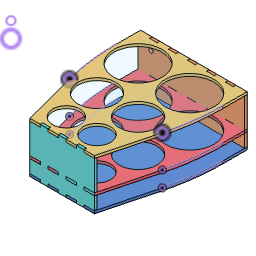
Zip Ties Peg Board Holder Laser Cut Version v5 (Autodesk Fusion 360 design; units mm, degrees)
Autodesk Fusion 360 part; units mm, degrees
sketch "Sketch1" plane through (0, 0, 0) normal (0, 1, 0) x (1, 0, 0) in component "Top Part"
  line L0 (0, 0) -> (24.5, 0) construction
  circle A0 centre (24.5, 0) radius 22.5
  line L1 (0, 0) -> (0, 91) construction
  circle A1 centre (30.75, 55.25) radius 28.75
  circle A2 centre (18.25, -42.75) radius 16.25
  line L2 (0, -66) -> (38.5, -66)
  line L3 (0, 91) -> (63.5, 91)
  line L4 (63.5, 91) -> (63.5, 29.5)
  line L5 (38.5, -66) -> (63.5, 29.5)
  line L6 (0, 91) -> (-63.5, 91)
  line L7 (-63.5, 91) -> (-63.5, 29.5)
  line L8 (-38.5, -66) -> (-63.5, 29.5)
  line L9 (0, -66) -> (-38.5, -66)
  circle A3 centre (-30.75, 55.25) radius 28.75
  circle A4 centre (-24.5, 0) radius 22.5
  circle A5 centre (-18.25, -42.75) radius 16.25
  line L10 (40.8333, 91) -> (49.8333, 91)
  line L11 (49.8333, 91) -> (49.8333, 88)
  line L12 (49.8333, 88) -> (40.8333, 88)
  line L13 (40.8333, 88) -> (40.8333, 91)
  line L14 (27.1667, 91) -> (18.1667, 91)
  line L15 (18.1667, 91) -> (18.1667, 88)
  line L16 (18.1667, 88) -> (27.1667, 88)
  line L17 (27.1667, 88) -> (27.1667, 91)
  line L18 (27.1667, 89.5) -> (40.8333, 89.5) construction
  line L19 (0, 91) -> (4.5, 91)
  line L20 (4.5, 91) -> (4.5, 88)
  line L21 (4.5, 88) -> (0, 88)
  line L22 (4.5, 89.5) -> (18.1667, 89.5) construction
  line L23 (49.8333, 89.5) -> (63.5, 89.5) construction
  line L24 (-49.8333, 91) -> (-49.8333, 88)
  line L25 (-49.8333, 88) -> (-40.8333, 88)
  line L26 (-40.8333, 88) -> (-40.8333, 91)
  line L27 (-27.1667, 88) -> (-27.1667, 91)
  line L28 (-18.1667, 88) -> (-27.1667, 88)
  line L29 (-18.1667, 91) -> (-18.1667, 88)
  line L30 (-4.5, 91) -> (-4.5, 88)
  line L31 (-4.5, 88) -> (0, 88)
  line L32 (0, -66) -> (4.5, -66)
  line L33 (4.5, -66) -> (4.5, -63)
  line L34 (4.5, -63) -> (0, -63)
  line L35 (17, -66) -> (26, -66)
  line L36 (26, -66) -> (26, -63)
  line L37 (26, -63) -> (17, -63)
  line L38 (17, -63) -> (17, -66)
  line L39 (38.5, -66) -> (38.5, -62) construction
  line L40 (26, -64.5) -> (38.5, -64.5) construction
  line L41 (17, -64.5) -> (4.5, -64.5) construction
  line L42 (-26, -66) -> (-26, -63)
  line L43 (-26, -63) -> (-17, -63)
  line L44 (-17, -63) -> (-17, -66)
  line L45 (-4.5, -66) -> (-4.5, -63)
  line L46 (-4.5, -63) -> (0, -63)
  dimension "d6" = 24.5
  dimension "d7" = 45
  dimension "d8" = 57.5
  dimension "d9" = 55.25
  dimension "d10" = 30.75
  dimension "d11" = 32.5
  dimension "d12" = 42.75
  dimension "d13" = 18.25
  dimension "d14" = 23.25
  dimension "d15" = 38.5
  dimension "d16" = 63.5
  dimension "d17" = 35.75
  dimension "d18" = 61.5
  dimension "d21" = 3
  dimension "d22" = 9
  dimension "d23" = 9
  dimension "d24" = 3
  dimension "d25" = 4.5
  dimension "d26" = 3
  dimension "d27" = 4.5
  dimension "d28" = 3
  dimension "d29" = 3
  dimension "d30" = 9
  constraint coincident L0.start L1.start
  constraint horizontal L0
  constraint coincident L0.end A0.centre
  constraint perpendicular L0 L1
  constraint horizontal L2
  constraint horizontal L3
  constraint perpendicular L3 L4
  constraint symmetric A0 L1 A4
  constraint symmetric L1 A1 A3
  constraint symmetric L1 A2 A5
  constraint symmetric L1 L2.start L9.start
  constraint symmetric L1 L2.end L8.start
  constraint symmetric L1 L3.start L6.start
  constraint symmetric L1 L3.end L6.end
  constraint symmetric L1 L4.end L7.end
  constraint horizontal L10
  constraint vertical L11
  constraint horizontal L12
  constraint vertical L13
  constraint coincident L3 L10.start
  constraint horizontal L14
  constraint vertical L15
  constraint horizontal L16
  constraint vertical L17
  constraint coincident L3 L14.start
  constraint coincident L1.end L3.start
  constraint midpoint L17 L18.start
  constraint midpoint L13 L18.end
  constraint horizontal L19
  constraint vertical L20
  constraint horizontal L21
  constraint midpoint L20 L22.start
  constraint midpoint L15 L22.end
  constraint midpoint L11 L23.start
  constraint coincident L4 L23.end
  constraint perpendicular L4 L23
  constraint equal L18 L23
  constraint equal L18 L22
  constraint symmetric L1 L10.start L26.end
  constraint symmetric L1 L10.end L24.start
  constraint symmetric L1 L11.end L24.end
  constraint symmetric L1 L12.end L25.end
  constraint symmetric L1 L14.start L27.end
  constraint symmetric L1 L14.end L29.start
  constraint symmetric L1 L15.end L28.start
  constraint symmetric L1 L16.end L27.start
  constraint symmetric L1 L19.end L30.start
  constraint symmetric L1 L20.end L30.end
  constraint symmetric L1 L21.end L31.end
  constraint coincident L2.start L9.start
  constraint horizontal L32
  constraint vertical L33
  constraint horizontal L34
  constraint horizontal L35
  constraint vertical L36
  constraint horizontal L37
  constraint vertical L38
  constraint coincident L2 L35.start
  constraint perpendicular L2 L39
  constraint midpoint L36 L40.start
  constraint coincident L39 L40.end
  constraint perpendicular L39 L40
  constraint midpoint L38 L41.start
  constraint midpoint L33 L41.end
  constraint equal L40 L41
  constraint symmetric L1 L32.end L45.start
  constraint symmetric L1 L33.end L45.end
  constraint symmetric L1 L34.end L46.end
  constraint symmetric L1 L35.start L44.end
  constraint symmetric L1 L35.end L42.start
  constraint symmetric L1 L36.end L42.end
  constraint symmetric L1 L37.end L43.end
  measures "d6" distance of L0.start L0.end
  measures "d7" diameter of A0
  measures "d8" diameter of A1
  measures "d9" vertical distance of L0.end A1.centre
  measures "d10" distance of L1 A1.centre
  measures "d11" diameter of A2
  measures "d12" vertical distance of L0.end A2.centre
  measures "d13" distance of L1 A2.centre
  measures "d14" distance of A2.centre L2
  measures "d15" distance of L2.start L2.end
  measures "d16" distance of L1.end L3.end
  measures "d17" distance of A1.centre L3
  measures "d18" distance of L3.end L4.end
  measures "d21" distance of L3 L12
  measures "d22" distance of L11.end L12.end
  measures "d23" distance of L15.end L16.end
  measures "d24" distance of L14 L16
  measures "d25" distance of L1 L20
  measures "d26" distance of L19 L21
  measures "d27" distance of L33.end L34.end
  measures "d28" distance of L32.end L33.end
  measures "d29" distance of L35.start L37.end
  measures "d30" distance of L36.end L37.end
extrude "Extrude1" add sketch "Sketch1" along normal blind 3 contours L2 L3 L4 L5 L6 L7 L8 L9 L11 L12 L13 L15 L16 L17 L20 L21 L24 L25 L26 L27 L28 L29 L30 L31 L33 L34 L36 L37 L38 L42 L43 L44 L45 L46 makes body 1 in component "Top Part"
sketch "Sketch1 (2)" plane through (0, 0, 66) normal (0, 0, 1) x (1, 0, 0) in component "Front Part"
  line L0 (-38.5, 0) -> (-26, 0)
  line L1 (-26, 0) -> (-26, 3)
  line L2 (-26, 3) -> (-38.5, 3)
  line L3 (-38.5, 3) -> (-38.5, 0)
  line L4 (-26, 0) -> (-17, 0)
  line L5 (-26, 0) -> (-17, 0)
  line L6 (-17, 0) -> (-17, 3)
  line L7 (-17, 3) -> (-26, 3)
  line L8 (-26, 3) -> (-26, 0)
  line L9 (-17, 0) -> (-4.5, 0)
  line L10 (-4.5, 0) -> (-4.5, 3)
  line L11 (-4.5, 3) -> (-17, 3)
  line L12 (-17, 3) -> (-17, 0)
  line L13 (-4.5, 3) -> (4.5, 3)
  line L14 (-4.5, 0) -> (4.5, 0)
  line L15 (4.5, 0) -> (4.5, 3)
  line L16 (4.5, 3) -> (-4.5, 3)
  line L17 (-4.5, 3) -> (-4.5, 0)
  line L18 (4.5, 3) -> (17, 3)
  line L19 (4.5, 0) -> (17, 0)
  line L20 (17, 0) -> (17, 3)
  line L21 (17, 3) -> (4.5, 3)
  line L22 (4.5, 3) -> (4.5, 0)
  line L23 (26, 0) -> (17, 0)
  line L24 (17, 0) -> (26, 0)
  line L25 (26, 0) -> (26, 3)
  line L26 (26, 3) -> (17, 3)
  line L27 (17, 3) -> (17, 0)
  line L28 (26, 0) -> (38.5, 0)
  line L29 (38.5, 0) -> (38.5, 3)
  line L30 (38.5, 3) -> (26, 3)
  line L31 (26, 3) -> (26, 0)
  line L32 (-38.5, 3) -> (38.5, 3)
  line L33 (38.5, 3) -> (38.5, -57)
  line L34 (38.5, -57) -> (-38.5, -57)
  line L35 (-38.5, -57) -> (-38.5, 3)
  line L36 (-38.5, -27) -> (38.5, -27) construction
  line L37 (-38.5, -54) -> (-26, -54)
  line L38 (-26, -54) -> (-26, -57)
  line L39 (-17, -57) -> (-17, -54)
  line L40 (-17, -54) -> (-4.5, -54)
  line L41 (-4.5, -54) -> (-4.5, -57)
  line L42 (4.5, -57) -> (4.5, -54)
  line L43 (4.5, -54) -> (17, -54)
  line L44 (17, -57) -> (17, -54)
  line L45 (26, -54) -> (26, -57)
  line L46 (26, -54) -> (38.5, -54)
  dimension "d33" = 60
  constraint horizontal L32
  constraint vertical L33
  constraint horizontal L34
  constraint vertical L35
  constraint coincident L2.end L3.start
  constraint coincident L29.end L33
  constraint midpoint L35 L36.start
  constraint midpoint L33 L36.end
  constraint symmetric L0.start L36 L37.start
  constraint symmetric L0.end L36 L37.end
  constraint symmetric L1.end L36 L38.end
  constraint symmetric L4.end L36 L39.end
  constraint symmetric L9.end L36 L40.end
  constraint symmetric L10.end L36 L41.end
  constraint symmetric L6.end L36 L39.start
  constraint symmetric L14.end L36 L42.end
  constraint symmetric L19.end L36 L43.end
  constraint symmetric L13.end L36 L42.start
  constraint symmetric L23.start L36 L45.start
  constraint symmetric L25.end L36 L45.end
  constraint symmetric L18.end L36 L44.start
  constraint symmetric L28.end L36 L46.end
  measures "d33" distance of L29.end L33.end
extrude "Extrude1'" add sketch "Sketch1 (2)" against normal blind 3 separate body contours L0 L4 L5 L9 L14 L19 L23 L24 L28 L33 L34 L35 L37 L38 L39 L40 L41 L42 L43 L44 L45 L46 | L1 L4 L5 L6 L7 L8 L12 L32 | L10 L13 L14 L15 L16 L17 L22 L32 | L20 L23 L24 L25 L26 L27 L31 L32 makes body 2 in component "Front Part"
sketch "Sketch1 (3)" plane through (0, 0, -91) normal (0, 0, -1) x (-1, 0, 0) in component "Back Part"
  line L0 (-18.1667, 0) -> (-4.5, 0)
  line L1 (-4.5, 0) -> (-4.5, 3)
  line L2 (-4.5, 3) -> (-18.1667, 3)
  line L3 (-18.1667, 3) -> (-18.1667, 0)
  line L4 (-63.5, 0) -> (-49.8333, 0)
  line L5 (-49.8333, 0) -> (-49.8333, 3)
  line L6 (-49.8333, 3) -> (-63.5, 3)
  line L7 (-63.5, 3) -> (-63.5, 0)
  line L8 (-49.8333, 0) -> (-40.8333, 0)
  line L9 (-40.8333, 0) -> (-40.8333, 3)
  line L10 (-40.8333, 3) -> (-49.8333, 3)
  line L11 (-49.8333, 3) -> (-49.8333, 0)
  line L12 (-40.8333, 0) -> (-27.1667, 0)
  line L13 (-27.1667, 0) -> (-27.1667, 3)
  line L14 (-27.1667, 3) -> (-40.8333, 3)
  line L15 (-40.8333, 3) -> (-40.8333, 0)
  line L16 (-27.1667, 0) -> (-18.1667, 0)
  line L17 (-18.1667, 0) -> (-18.1667, 3)
  line L18 (-18.1667, 3) -> (-27.1667, 3)
  line L19 (-27.1667, 3) -> (-27.1667, 0)
  line L20 (-4.5, 0) -> (4.5, 0)
  line L21 (4.5, 0) -> (4.5, 3)
  line L22 (4.5, 3) -> (-4.5, 3)
  line L23 (-4.5, 3) -> (-4.5, 0)
  line L24 (4.5, 0) -> (18.1667, 0)
  line L25 (18.1667, 0) -> (18.1667, 3)
  line L26 (18.1667, 3) -> (4.5, 3)
  line L27 (4.5, 3) -> (4.5, 0)
  line L28 (18.1667, 0) -> (27.1667, 0)
  line L29 (27.1667, 0) -> (27.1667, 3)
  line L30 (27.1667, 3) -> (18.1667, 3)
  line L31 (18.1667, 3) -> (18.1667, 0)
  line L32 (27.1667, 0) -> (40.8333, 0)
  line L33 (40.8333, 0) -> (40.8333, 3)
  line L34 (40.8333, 3) -> (27.1667, 3)
  line L35 (27.1667, 3) -> (27.1667, 0)
  line L36 (40.8333, 0) -> (49.8333, 0)
  line L37 (49.8333, 0) -> (49.8333, 3)
  line L38 (49.8333, 3) -> (40.8333, 3)
  line L39 (40.8333, 3) -> (40.8333, 0)
  line L40 (49.8333, 0) -> (63.5, 0)
  line L41 (63.5, 0) -> (63.5, 3)
  line L42 (63.5, 3) -> (49.8333, 3)
  line L43 (49.8333, 3) -> (49.8333, 0)
  line L44 (-63.5, 3) -> (63.5, 3)
  line L45 (63.5, 3) -> (63.5, -57)
  line L46 (63.5, -57) -> (-63.5, -57)
  line L47 (-63.5, -57) -> (-63.5, 3)
  line L48 (-63.5, -27) -> (63.5, -27) construction
  line L49 (-63.5, -54) -> (-49.8333, -54)
  line L50 (-49.8333, -54) -> (-49.8333, -57)
  line L51 (-40.8333, -54) -> (-40.8333, -57)
  line L52 (-40.8333, -54) -> (-27.1667, -54)
  line L53 (-27.1667, -57) -> (-27.1667, -54)
  line L54 (-18.1667, -57) -> (-18.1667, -54)
  line L55 (-18.1667, -54) -> (-4.5, -54)
  line L56 (-4.5, -57) -> (-4.5, -54)
  line L57 (4.5, -54) -> (4.5, -57)
  line L58 (4.5, -54) -> (18.1667, -54)
  line L59 (18.1667, -57) -> (18.1667, -54)
  line L60 (27.1667, -54) -> (27.1667, -57)
  line L61 (27.1667, -54) -> (40.8333, -54)
  line L62 (40.8333, -57) -> (40.8333, -54)
  line L63 (49.8333, -54) -> (49.8333, -57)
  line L64 (49.8333, -54) -> (63.5, -54)
  circle A0 centre (-48, -9) radius 2.5
  line L65 (-26, -54) -> (-26, -57)
  line L66 (-26, -57) -> (-17, -57)
  line L67 (-17, -57) -> (-17, -54)
  line L68 (-17, -54) -> (-4.5, -54)
  line L69 (-4.5, -54) -> (-4.5, -57)
  line L70 (-4.5, -57) -> (4.5, -57)
  line L71 (4.5, -57) -> (4.5, -54)
  line L72 (4.5, -54) -> (17, -54)
  line L73 (17, -54) -> (17, -57)
  line L74 (17, -57) -> (26, -57)
  line L75 (26, -57) -> (26, -54)
  line L76 (26, -54) -> (38.5, -54)
  line L77 (38.5, -54) -> (38.5, 0)
  line L78 (38.5, 0) -> (26, 0)
  line L79 (26, 0) -> (26, 3)
  line L80 (26, 3) -> (17, 3)
  line L81 (17, 3) -> (17, 0)
  line L82 (17, 0) -> (4.5, 0)
  line L83 (4.5, 0) -> (4.5, 3)
  line L84 (4.5, 3) -> (-4.5, 3)
  line L85 (-4.5, 3) -> (-4.5, 0)
  line L86 (-4.5, 0) -> (-17, 0)
  line L87 (-17, 0) -> (-17, 3)
  line L88 (-17, 3) -> (-26, 3)
  line L89 (-26, 3) -> (-26, 0)
  line L90 (-26, 0) -> (-38.5, 0)
  line L91 (-38.5, 0) -> (-38.5, -54)
  line L92 (-38.5, -54) -> (-26, -54)
  circle A1 centre (48, -9) radius 2.5
  line L93 (48, -9) -> (63.5, -9) construction
  line L94 (-48, -9) -> (-63.5, -9) construction
  circle A2 centre (-48, -45) radius 2.5
  circle A3 centre (48, -45) radius 2.5
  dimension "d36" = 60
  dimension "d46" = 5
  dimension "d48" = 5
  dimension "d49" = 96
  dimension "d50" = 36
  constraint horizontal L44
  constraint vertical L45
  constraint horizontal L46
  constraint vertical L47
  constraint coincident L6.end L7.start
  constraint coincident L41.end L45
  constraint midpoint L47 L48.start
  constraint midpoint L45 L48.end
  constraint symmetric L0.start L48 L54.end
  constraint symmetric L0.end L48 L55.end
  constraint symmetric L2.end L48 L54.start
  constraint symmetric L4.start L48 L49.start
  constraint symmetric L4.end L48 L49.end
  constraint symmetric L5.end L48 L50.end
  constraint symmetric L8.end L48 L51.start
  constraint symmetric L9.end L48 L51.end
  constraint symmetric L12.end L48 L52.end
  constraint symmetric L13.end L48 L53.start
  constraint symmetric L20.end L48 L57.start
  constraint symmetric L21.end L48 L57.end
  constraint symmetric L1.end L48 L56.start
  constraint symmetric L24.end L48 L58.end
  constraint symmetric L28.end L48 L60.start
  constraint symmetric L29.end L48 L60.end
  constraint symmetric L25.end L48 L59.start
  constraint symmetric L32.end L48 L61.end
  constraint symmetric L36.end L48 L63.start
  constraint symmetric L37.end L48 L63.end
  constraint symmetric L33.end L48 L62.start
  constraint symmetric L40.end L48 L64.end
  constraint coincident A1.centre L93.start
  constraint coincident L45 L93.end
  constraint perpendicular L45 L93
  constraint coincident A0.centre L94.start
  constraint coincident L47 L94.end
  constraint perpendicular L47 L94
  constraint collinear L93 L94
  constraint equal L93 L94
  constraint symmetric L48 A0 A2
  constraint symmetric L48 A1 A3
  measures "d36" distance of L41.end L45.end
  measures "d46" diameter of A0
  measures "d48" diameter of A1
  measures "d49" distance of A0.centre A1.centre
  measures "d50" distance of A1.centre A3.centre
extrude "Extrude1''" add sketch "Sketch1 (3)" against normal blind 3 separate body contours L3 L16 L17 L18 L44 L88 L89 | L0 L12 L16 L20 L24 L28 L32 L46 L52 L54 L55 L56 L57 L58 L59 L61 L65 L66 L68 L69 L70 L71 L72 L74 L75 L76 L77 L78 L82 L86 L90 L91 L92 | L13 L16 L18 L19 L44 L89 L90 | L1 L20 L21 L22 L23 L27 L44 L83 L84 L85 | L4 L8 L12 L46 L47 L49 L50 L51 L52 L91 | L5 L8 L9 L10 L11 L15 L44 | L25 L28 L30 L31 L44 L79 L80 | L46 L53 L65 L92 | L28 L29 L30 L35 L44 L78 L79 | L32 L36 L40 L45 L46 L61 L62 L63 L64 L77 | L33 L36 L37 L38 L39 L43 L44 | L46 L60 L75 L76 makes body 3 in component "Back Part"
sketch "Sketch1 (4)" plane through (0, -57, 0) normal (0, -1, 0) x (1, 0, 0) in component "Bottom Part"
  line L0 (40.8333, -91) -> (49.8333, -91)
  line L1 (49.8333, -91) -> (49.8333, -88)
  line L2 (49.8333, -88) -> (40.8333, -88)
  line L3 (40.8333, -88) -> (40.8333, -91)
  line L4 (49.8333, -91) -> (63.5, -91)
  line L5 (63.5, -91) -> (63.5, -88)
  line L6 (63.5, -88) -> (49.8333, -88)
  line L7 (49.8333, -88) -> (49.8333, -91)
  line L8 (27.1667, -91) -> (40.8333, -91)
  line L9 (40.8333, -91) -> (40.8333, -88)
  line L10 (40.8333, -88) -> (27.1667, -88)
  line L11 (27.1667, -88) -> (27.1667, -91)
  line L12 (18.1667, -91) -> (27.1667, -91)
  line L13 (27.1667, -91) -> (27.1667, -88)
  line L14 (27.1667, -88) -> (18.1667, -88)
  line L15 (18.1667, -88) -> (18.1667, -91)
  line L16 (4.5, -91) -> (18.1667, -91)
  line L17 (18.1667, -91) -> (18.1667, -88)
  line L18 (18.1667, -88) -> (4.5, -88)
  line L19 (4.5, -88) -> (4.5, -91)
  line L20 (-4.5, -91) -> (4.5, -91)
  line L21 (4.5, -91) -> (4.5, -88)
  line L22 (4.5, -88) -> (-4.5, -88)
  line L23 (-4.5, -88) -> (-4.5, -91)
  line L24 (-18.1667, -91) -> (-4.5, -91)
  line L25 (-4.5, -91) -> (-4.5, -88)
  line L26 (-4.5, -88) -> (-18.1667, -88)
  line L27 (-18.1667, -88) -> (-18.1667, -91)
  line L28 (-27.1667, -91) -> (-18.1667, -91)
  line L29 (-18.1667, -91) -> (-18.1667, -88)
  line L30 (-18.1667, -88) -> (-27.1667, -88)
  line L31 (-27.1667, -88) -> (-27.1667, -91)
  line L32 (-40.8333, -91) -> (-27.1667, -91)
  line L33 (-27.1667, -91) -> (-27.1667, -88)
  line L34 (-27.1667, -88) -> (-40.8333, -88)
  line L35 (-40.8333, -88) -> (-40.8333, -91)
  line L36 (-49.8333, -91) -> (-40.8333, -91)
  line L37 (-40.8333, -91) -> (-40.8333, -88)
  line L38 (-40.8333, -88) -> (-49.8333, -88)
  line L39 (-49.8333, -88) -> (-49.8333, -91)
  line L40 (-63.5, -91) -> (-49.8333, -91)
  line L41 (-49.8333, -91) -> (-49.8333, -88)
  line L42 (-49.8333, -88) -> (-63.5, -88)
  line L43 (-63.5, -88) -> (-63.5, -91)
  circle A0 centre (24.5, 0) radius 22.5
  circle A1 centre (-30.75, -55.25) radius 28.75
  circle A2 centre (-24.5, 0) radius 22.5
  circle A3 centre (30.75, -55.25) radius 28.75
  circle A4 centre (-18.25, 42.75) radius 16.25
  circle A5 centre (18.25, 42.75) radius 16.25
  line L44 (-4.5, 63) -> (-4.5, 66)
  line L45 (-4.5, 66) -> (-17, 66)
  line L46 (-17, 66) -> (-17, 63)
  line L47 (-17, 63) -> (-26, 63)
  line L48 (-26, 63) -> (-26, 66)
  line L49 (-26, 66) -> (-38.5, 66)
  line L50 (-38.5, 66) -> (-63.5, -29.5)
  line L51 (-63.5, -29.5) -> (-63.5, -91)
  line L52 (-63.5, -91) -> (-49.8333, -91)
  line L53 (-49.8333, -91) -> (-49.8333, -88)
  line L54 (-49.8333, -88) -> (-40.8333, -88)
  line L55 (-40.8333, -88) -> (-40.8333, -91)
  line L56 (-40.8333, -91) -> (-27.1667, -91)
  line L57 (-27.1667, -91) -> (-27.1667, -88)
  line L58 (-27.1667, -88) -> (-18.1667, -88)
  line L59 (-18.1667, -88) -> (-18.1667, -91)
  line L60 (-18.1667, -91) -> (-4.5, -91)
  line L61 (-4.5, -91) -> (-4.5, -88)
  line L62 (-4.5, -88) -> (4.5, -88)
  line L63 (4.5, -88) -> (4.5, -91)
  line L64 (4.5, -91) -> (18.1667, -91)
  line L65 (18.1667, -91) -> (18.1667, -88)
  line L66 (18.1667, -88) -> (27.1667, -88)
  line L67 (27.1667, -88) -> (27.1667, -91)
  line L68 (27.1667, -91) -> (40.8333, -91)
  line L69 (40.8333, -91) -> (40.8333, -88)
  line L70 (40.8333, -88) -> (49.8333, -88)
  line L71 (49.8333, -88) -> (49.8333, -91)
  line L72 (49.8333, -91) -> (63.5, -91)
  line L73 (63.5, -91) -> (63.5, -29.5)
  line L74 (63.5, -29.5) -> (38.5, 66)
  line L75 (38.5, 66) -> (26, 66)
  line L76 (26, 66) -> (26, 63)
  line L77 (26, 63) -> (17, 63)
  line L78 (17, 63) -> (17, 66)
  line L79 (17, 66) -> (4.5, 66)
  line L80 (4.5, 66) -> (4.5, 63)
  line L81 (4.5, 63) -> (-4.5, 63)
  line L82 (26, 66) -> (38.5, 66)
  line L83 (38.5, 66) -> (26, 66)
  line L84 (26, 66) -> (26, 63)
  line L85 (26, 63) -> (38.5, 63)
  line L86 (38.5, 63) -> (38.5, 66)
  line L87 (26, 66) -> (17, 66)
  line L88 (17, 66) -> (17, 63)
  line L89 (17, 63) -> (26, 63)
  line L90 (26, 63) -> (26, 66)
  line L91 (17, 66) -> (4.5, 66)
  line L92 (4.5, 66) -> (4.5, 63)
  line L93 (4.5, 63) -> (17, 63)
  line L94 (17, 63) -> (17, 66)
  line L95 (4.5, 66) -> (-4.5, 66)
  line L96 (-4.5, 66) -> (-4.5, 63)
  line L97 (-4.5, 63) -> (4.5, 63)
  line L98 (4.5, 63) -> (4.5, 66)
  line L99 (-4.5, 66) -> (-17, 66)
  line L100 (-17, 66) -> (-17, 63)
  line L101 (-17, 63) -> (-4.5, 63)
  line L102 (-4.5, 63) -> (-4.5, 66)
  line L103 (-17, 66) -> (-26, 66)
  line L104 (-26, 66) -> (-26, 63)
  line L105 (-26, 63) -> (-17, 63)
  line L106 (-17, 63) -> (-17, 66)
  line L107 (-26, 66) -> (-38.5, 66)
  line L108 (-38.5, 66) -> (-38.5, 63)
  line L109 (-38.5, 63) -> (-26, 63)
  line L110 (-26, 63) -> (-26, 66)
extrude "Extrude1'''" add sketch "Sketch1 (4)" against normal blind 3 separate body contours L3 L8 L9 L10 L11 L13 L67 L68 L69 | L1 L4 L5 L6 L7 L71 L72 L73 | L2 L6 L10 L14 L18 L22 L26 L30 L34 L38 L42 L47 L50 L51 L54 L58 L62 L66 L70 L73 L74 L77 L81 L85 L86 L89 L93 L97 L101 L105 L108 L109 | L15 L16 L17 L18 L19 L21 L63 L64 L65 | L23 L24 L25 L26 L27 L29 L59 L60 L61 | L75 L76 L82 L83 L84 L85 L86 L90 | L31 L32 L33 L34 L35 L37 L55 L56 L57 | L78 L79 L80 L88 L91 L92 L93 L94 L98 | L39 L40 L41 L42 L43 L51 L52 L53 | L44 L45 L46 L96 L99 L100 L101 L102 L106 | L48 L49 L104 L107 L108 L109 L110 | A0 | A1 | A2 | A3 | A4 | A5 makes body 4 in component "Bottom Part"
ref_plane "WorkPlane1" through (0, -37, -12.5) normal (0, -1, 0) x (1, 0, 0) in component "Middle Part"
sketch "Sketch1 (5)" plane through (0, -37, 0) normal (0, -1, 0) x (-1, 0, 0) in component "Middle Part"
  circle A0 centre (-24.5, 0) radius 22.5
  circle A1 centre (30.75, 55.25) radius 28.75
  circle A2 centre (24.5, 0) radius 22.5
  circle A3 centre (-30.75, 55.25) radius 28.75
  circle A4 centre (18.25, -42.75) radius 16.25
  circle A5 centre (-18.25, -42.75) radius 16.25
  line L0 (4.5, -63) -> (4.5, -66)
  line L1 (4.5, -66) -> (17, -66)
  line L2 (17, -66) -> (17, -63)
  line L3 (17, -63) -> (26, -63)
  line L4 (26, -63) -> (26, -66)
  line L5 (26, -66) -> (38.5, -66)
  line L6 (38.5, -66) -> (63.5, 29.5)
  line L7 (63.5, 29.5) -> (63.5, 91)
  line L8 (63.5, 91) -> (49.8333, 91)
  line L9 (49.8333, 91) -> (49.8333, 88)
  line L10 (49.8333, 88) -> (40.8333, 88)
  line L11 (40.8333, 88) -> (40.8333, 91)
  line L12 (40.8333, 91) -> (27.1667, 91)
  line L13 (27.1667, 91) -> (27.1667, 88)
  line L14 (27.1667, 88) -> (18.1667, 88)
  line L15 (18.1667, 88) -> (18.1667, 91)
  line L16 (18.1667, 91) -> (4.5, 91)
  line L17 (4.5, 91) -> (4.5, 88)
  line L18 (4.5, 88) -> (-4.5, 88)
  line L19 (-4.5, 88) -> (-4.5, 91)
  line L20 (-4.5, 91) -> (-18.1667, 91)
  line L21 (-18.1667, 91) -> (-18.1667, 88)
  line L22 (-18.1667, 88) -> (-27.1667, 88)
  line L23 (-27.1667, 88) -> (-27.1667, 91)
  line L24 (-27.1667, 91) -> (-40.8333, 91)
  line L25 (-40.8333, 91) -> (-40.8333, 88)
  line L26 (-40.8333, 88) -> (-49.8333, 88)
  line L27 (-49.8333, 88) -> (-49.8333, 91)
  line L28 (-49.8333, 91) -> (-63.5, 91)
  line L29 (-63.5, 91) -> (-63.5, 29.5)
  line L30 (-63.5, 29.5) -> (-38.5, -66)
  line L31 (-38.5, -66) -> (-26, -66)
  line L32 (-26, -66) -> (-26, -63)
  line L33 (-26, -63) -> (-17, -63)
  line L34 (-17, -63) -> (-17, -66)
  line L35 (-17, -66) -> (-4.5, -66)
  line L36 (-4.5, -66) -> (-4.5, -63)
  line L37 (-4.5, -63) -> (4.5, -63)
extrude "Extrude1''''" add sketch "Sketch1 (5)" along normal mid plane 3 separate body makes body 5 in component "Middle Part"
fillet "Fillet1" radius 252.5 2 edges at (-63.5, 1.5, -29.5) (63.5, 1.5, -29.5) on bodies 1 in component "Top Part"
fillet "Fillet1'" radius 252.5 2 edges at (-63.5, -37, -29.5) (63.5, -37, -29.5) on bodies 5 in component "Middle Part"
fillet "Fillet1''" radius 252.5 2 edges at (-63.5, -55.5, -29.5) (63.5, -55.5, -29.5) on bodies 4 in component "Bottom Part"
sketch "Front Part DXF" plane through (0, 0, 66) normal (0, 0, 1) x (1, 0, 0)
  line L0 (26, -57) -> (26, -54)
  line L1 (26, -54) -> (38.5, -54)
  line L2 (38.5, -54) -> (38.5, 0)
  line L3 (38.5, 0) -> (26, 0)
  line L4 (26, 0) -> (26, 3)
  line L5 (26, 3) -> (17, 3)
  line L6 (17, 3) -> (17, 0)
  line L7 (17, 0) -> (4.5, 0)
  line L8 (4.5, 0) -> (4.5, 3)
  line L9 (4.5, 3) -> (-4.5, 3)
  line L10 (-4.5, 3) -> (-4.5, 0)
  line L11 (-4.5, 0) -> (-17, 0)
  line L12 (-17, 0) -> (-17, 3)
  line L13 (-17, 3) -> (-26, 3)
  line L14 (-26, 3) -> (-26, 0)
  line L15 (-26, 0) -> (-38.5, 0)
  line L16 (-38.5, 0) -> (-38.5, -54)
  line L17 (-38.5, -54) -> (-26, -54)
  line L18 (-26, -54) -> (-26, -57)
  line L19 (-26, -57) -> (-17, -57)
  line L20 (-17, -57) -> (-17, -54)
  line L21 (-17, -54) -> (-4.5, -54)
  line L22 (-4.5, -54) -> (-4.5, -57)
  line L23 (-4.5, -57) -> (4.5, -57)
  line L24 (4.5, -57) -> (4.5, -54)
  line L25 (4.5, -54) -> (17, -54)
  line L26 (17, -54) -> (17, -57)
  line L27 (17, -57) -> (26, -57)
sketch "Top Part DXF" plane through (0, 3, 0) normal (0, 1, 0) x (-1, 0, 0)
  circle A0 centre (-24.5, 0) radius 22.5
  circle A1 centre (30.75, -55.25) radius 28.75
  circle A2 centre (24.5, 0) radius 22.5
  circle A3 centre (-30.75, -55.25) radius 28.75
  circle A4 centre (18.25, 42.75) radius 16.25
  circle A5 centre (-18.25, 42.75) radius 16.25
  line L0 (4.5, 66) -> (4.5, 63)
  line L1 (4.5, 63) -> (-4.5, 63)
  line L2 (-4.5, 63) -> (-4.5, 66)
  line L3 (-4.5, 66) -> (-17, 66)
  line L4 (-17, 66) -> (-17, 63)
  line L5 (-17, 63) -> (-26, 63)
  line L6 (-26, 63) -> (-26, 66)
  line L7 (-26, 66) -> (-38.5, 66)
  line L8 (-38.5, 66) -> (-55.2689, 1.9426)
  line L9 (-63.5, -62.0021) -> (-63.5, -91)
  line L10 (-63.5, -91) -> (-49.8333, -91)
  line L11 (-49.8333, -91) -> (-49.8333, -88)
  line L12 (-49.8333, -88) -> (-40.8333, -88)
  line L13 (-40.8333, -88) -> (-40.8333, -91)
  line L14 (-40.8333, -91) -> (-27.1667, -91)
  line L15 (-27.1667, -91) -> (-27.1667, -88)
  line L16 (-27.1667, -88) -> (-18.1667, -88)
  line L17 (-18.1667, -88) -> (-18.1667, -91)
  line L18 (-18.1667, -91) -> (-4.5, -91)
  line L19 (-4.5, -91) -> (-4.5, -88)
  line L20 (-4.5, -88) -> (4.5, -88)
  line L21 (4.5, -88) -> (4.5, -91)
  line L22 (4.5, -91) -> (18.1667, -91)
  line L23 (18.1667, -91) -> (18.1667, -88)
  line L24 (18.1667, -88) -> (27.1667, -88)
  line L25 (27.1667, -88) -> (27.1667, -91)
  line L26 (27.1667, -91) -> (40.8333, -91)
  line L27 (40.8333, -91) -> (40.8333, -88)
  line L28 (40.8333, -88) -> (49.8333, -88)
  line L29 (49.8333, -88) -> (49.8333, -91)
  line L30 (49.8333, -91) -> (63.5, -91)
  line L31 (63.5, -91) -> (63.5, -62.0021)
  line L32 (55.2689, 1.9426) -> (38.5, 66)
  line L33 (38.5, 66) -> (26, 66)
  line L34 (26, 66) -> (26, 63)
  line L35 (26, 63) -> (17, 63)
  line L36 (17, 63) -> (17, 66)
  line L37 (17, 66) -> (4.5, 66)
  arc A6 (-55.2689, 1.9426) -> (-63.5, -62.0021) centre (189, -62.0021) ccw
  arc A7 (63.5, -62.0021) -> (55.2689, 1.9426) centre (-189, -62.0021) ccw
sketch "Back Part DXF" plane through (0, 0, -88) normal (0, 0, 1) x (1, 0, 0)
  circle A0 centre (-48, -45) radius 2.5
  circle A1 centre (48, -9) radius 2.5
  circle A2 centre (48, -45) radius 2.5
  circle A3 centre (-48, -9) radius 2.5
  line L0 (27.1667, -54) -> (40.8333, -54)
  line L1 (40.8333, -54) -> (40.8333, -57)
  line L2 (40.8333, -57) -> (49.8333, -57)
  line L3 (49.8333, -57) -> (49.8333, -54)
  line L4 (49.8333, -54) -> (63.5, -54)
  line L5 (63.5, -54) -> (63.5, 0)
  line L6 (63.5, 0) -> (49.8333, 0)
  line L7 (49.8333, 0) -> (49.8333, 3)
  line L8 (49.8333, 3) -> (40.8333, 3)
  line L9 (40.8333, 3) -> (40.8333, 0)
  line L10 (40.8333, 0) -> (27.1667, 0)
  line L11 (27.1667, 0) -> (27.1667, 3)
  line L12 (27.1667, 3) -> (18.1667, 3)
  line L13 (18.1667, 3) -> (18.1667, 0)
  line L14 (18.1667, 0) -> (4.5, 0)
  line L15 (4.5, 0) -> (4.5, 3)
  line L16 (4.5, 3) -> (-4.5, 3)
  line L17 (-4.5, 3) -> (-4.5, 0)
  line L18 (-4.5, 0) -> (-18.1667, 0)
  line L19 (-18.1667, 0) -> (-18.1667, 3)
  line L20 (-18.1667, 3) -> (-27.1667, 3)
  line L21 (-27.1667, 3) -> (-27.1667, 0)
  line L22 (-27.1667, 0) -> (-40.8333, 0)
  line L23 (-40.8333, 0) -> (-40.8333, 3)
  line L24 (-40.8333, 3) -> (-49.8333, 3)
  line L25 (-49.8333, 3) -> (-49.8333, 0)
  line L26 (-49.8333, 0) -> (-63.5, 0)
  line L27 (-63.5, 0) -> (-63.5, -54)
  line L28 (-63.5, -54) -> (-49.8333, -54)
  line L29 (-49.8333, -54) -> (-49.8333, -57)
  line L30 (-49.8333, -57) -> (-40.8333, -57)
  line L31 (-40.8333, -57) -> (-40.8333, -54)
  line L32 (-40.8333, -54) -> (-27.1667, -54)
  line L33 (-27.1667, -54) -> (-27.1667, -57)
  line L34 (-27.1667, -57) -> (-18.1667, -57)
  line L35 (-18.1667, -57) -> (-18.1667, -54)
  line L36 (-18.1667, -54) -> (-4.5, -54)
  line L37 (-4.5, -54) -> (-4.5, -57)
  line L38 (-4.5, -57) -> (4.5, -57)
  line L39 (4.5, -57) -> (4.5, -54)
  line L40 (4.5, -54) -> (18.1667, -54)
  line L41 (18.1667, -54) -> (18.1667, -57)
  line L42 (18.1667, -57) -> (27.1667, -57)
  line L43 (27.1667, -57) -> (27.1667, -54)
sketch "Middle Part DXF" plane through (0, -35.5, 0) normal (0, 1, 0) x (-1, 0, 0)
  circle A0 centre (-18.25, 42.75) radius 16.25
  circle A1 centre (24.5, 0) radius 22.5
  circle A2 centre (30.75, -55.25) radius 28.75
  circle A3 centre (-24.5, 0) radius 22.5
  circle A4 centre (-30.75, -55.25) radius 28.75
  circle A5 centre (18.25, 42.75) radius 16.25
  line L0 (4.5, 63) -> (-4.5, 63)
  line L1 (-4.5, 63) -> (-4.5, 66)
  line L2 (-4.5, 66) -> (-17, 66)
  line L3 (-17, 66) -> (-17, 63)
  line L4 (-17, 63) -> (-26, 63)
  line L5 (-26, 63) -> (-26, 66)
  line L6 (-26, 66) -> (-38.5, 66)
  line L7 (-38.5, 66) -> (-55.2689, 1.9426)
  line L8 (-63.5, -62.0021) -> (-63.5, -91)
  line L9 (-63.5, -91) -> (-49.8333, -91)
  line L10 (-49.8333, -91) -> (-49.8333, -88)
  line L11 (-49.8333, -88) -> (-40.8333, -88)
  line L12 (-40.8333, -88) -> (-40.8333, -91)
  line L13 (-40.8333, -91) -> (-27.1667, -91)
  line L14 (-27.1667, -91) -> (-27.1667, -88)
  line L15 (-27.1667, -88) -> (-18.1667, -88)
  line L16 (-18.1667, -88) -> (-18.1667, -91)
  line L17 (-18.1667, -91) -> (-4.5, -91)
  line L18 (-4.5, -91) -> (-4.5, -88)
  line L19 (-4.5, -88) -> (4.5, -88)
  line L20 (4.5, -88) -> (4.5, -91)
  line L21 (4.5, -91) -> (18.1667, -91)
  line L22 (18.1667, -91) -> (18.1667, -88)
  line L23 (18.1667, -88) -> (27.1667, -88)
  line L24 (27.1667, -88) -> (27.1667, -91)
  line L25 (27.1667, -91) -> (40.8333, -91)
  line L26 (40.8333, -91) -> (40.8333, -88)
  line L27 (40.8333, -88) -> (49.8333, -88)
  line L28 (49.8333, -88) -> (49.8333, -91)
  line L29 (49.8333, -91) -> (63.5, -91)
  line L30 (63.5, -91) -> (63.5, -62.0021)
  line L31 (55.2689, 1.9426) -> (38.5, 66)
  line L32 (38.5, 66) -> (26, 66)
  line L33 (26, 66) -> (26, 63)
  line L34 (26, 63) -> (17, 63)
  line L35 (17, 63) -> (17, 66)
  line L36 (17, 66) -> (4.5, 66)
  line L37 (4.5, 66) -> (4.5, 63)
  arc A6 (-55.2689, 1.9426) -> (-63.5, -62.0021) centre (189, -62.0021) ccw
  arc A7 (63.5, -62.0021) -> (55.2689, 1.9426) centre (-189, -62.0021) ccw
sketch "Bottom Part DXF" plane through (0, -54, 0) normal (0, 1, 0) x (-1, 0, 0)
  line L0 (26, 63) -> (17, 63)
  line L1 (17, 63) -> (17, 66)
  line L2 (17, 66) -> (4.5, 66)
  line L3 (4.5, 66) -> (4.5, 63)
  line L4 (4.5, 63) -> (-4.5, 63)
  line L5 (-4.5, 63) -> (-4.5, 66)
  line L6 (-4.5, 66) -> (-17, 66)
  line L7 (-17, 66) -> (-17, 63)
  line L8 (-17, 63) -> (-26, 63)
  line L9 (-26, 63) -> (-26, 66)
  line L10 (-26, 66) -> (-38.5, 66)
  line L11 (-38.5, 66) -> (-55.2689, 1.9426)
  line L12 (-63.5, -62.0021) -> (-63.5, -91)
  line L13 (-63.5, -91) -> (-49.8333, -91)
  line L14 (-49.8333, -91) -> (-49.8333, -88)
  line L15 (-49.8333, -88) -> (-40.8333, -88)
  line L16 (-40.8333, -88) -> (-40.8333, -91)
  line L17 (-40.8333, -91) -> (-27.1667, -91)
  line L18 (-27.1667, -91) -> (-27.1667, -88)
  line L19 (-27.1667, -88) -> (-18.1667, -88)
  line L20 (-18.1667, -88) -> (-18.1667, -91)
  line L21 (-18.1667, -91) -> (-4.5, -91)
  line L22 (-4.5, -91) -> (-4.5, -88)
  line L23 (-4.5, -88) -> (4.5, -88)
  line L24 (4.5, -88) -> (4.5, -91)
  line L25 (4.5, -91) -> (18.1667, -91)
  line L26 (18.1667, -91) -> (18.1667, -88)
  line L27 (18.1667, -88) -> (27.1667, -88)
  line L28 (27.1667, -88) -> (27.1667, -91)
  line L29 (27.1667, -91) -> (40.8333, -91)
  line L30 (40.8333, -91) -> (40.8333, -88)
  line L31 (40.8333, -88) -> (49.8333, -88)
  line L32 (49.8333, -88) -> (49.8333, -91)
  line L33 (49.8333, -91) -> (63.5, -91)
  line L34 (63.5, -91) -> (63.5, -62.0021)
  line L35 (55.2689, 1.9426) -> (38.5, 66)
  line L36 (38.5, 66) -> (26, 66)
  line L37 (26, 66) -> (26, 63)
  arc A0 (-55.2689, 1.9426) -> (-63.5, -62.0021) centre (189, -62.0021) ccw
  arc A1 (63.5, -62.0021) -> (55.2689, 1.9426) centre (-189, -62.0021) ccw
component "Top Part" placed x (1, 0, 0) y (0, 1, 0) z (0, 0, 1) at (0, 0, 0)
component "Front Part" placed x (1, 0, 0) y (0, 1, 0) z (0, 0, 1) at (0, 0, 0)
component "Back Part" placed x (1, 0, 0) y (0, 1, 0) z (0, 0, 1) at (0, 0, 0)
component "Bottom Part" placed x (1, 0, 0) y (0, 1, 0) z (0, 0, 1) at (0, 0, 0)
component "Middle Part" placed x (1, 0, 0) y (0, 1, 0) z (0, 0, 1) at (0, 0, 0)
equation "large = 57.5 mm"
equation "medium = 45 mm"
equation "small = 32.5 mm"
equation "spacing = 4 mm"
equation "height = 60 mm"
equation "d6 = spacing / 2 + medium / 2"
equation "d7 = medium"
equation "d8 = large"
equation "d9 = spacing + medium / 2 + large / 2"
equation "d10 = spacing / 2 + large / 2"
equation "d11 = small"
equation "d12 = spacing + small / 2 + medium / 2"
equation "d13 = small / 2 + spacing / 2"
equation "d14 = small / 2 + spacing + material_thickness"
equation "d15 = spacing / 2 + small + spacing"
equation "d16 = spacing / 2 + large + spacing"
equation "d17 = large / 2 + spacing + material_thickness"
equation "d18 = large + spacing"
equation "material_thickness = 3 mm"
equation "material_finger_width = 3 * material_thickness"
equation "d21 = material_thickness"
equation "d22 = material_finger_width"
equation "d23 = material_finger_width"
equation "d24 = material_thickness"
equation "d25 = material_finger_width / 2"
equation "d26 = material_thickness"
equation "d27 = material_finger_width / 2"
equation "d28 = material_thickness"
equation "d29 = material_thickness"
equation "d30 = material_finger_width"
equation "d31 = material_thickness"
equation "d33 = height"
equation "d34 = -material_thickness"
equation "d36 = height"
equation "d37 = -material_thickness"
equation "d39 = -material_thickness"
equation "middle_part_height_from_bottom = height / 3"
equation "d42 = -middle_part_height_from_bottom"
equation "d43 = material_thickness / 2"
equation "pegboard_hole_distance = 12 mm"
equation "d46 = pegboard_hole_dia"
equation "pegboard_hole_dia = 5 mm"
equation "d48 = pegboard_hole_dia"
equation "d49 = pegboard_hole_distance * 8"
equation "d50 = pegboard_hole_distance * 3"
named bodies: "Top Part"
